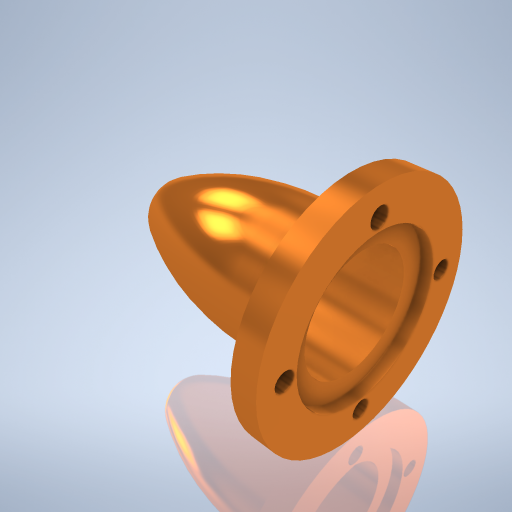
# Autodesk Inventor part: heizrohr
Saved by Autodesk Inventor 2024.2 (Build 282272000, 272)
## iProperties
Created: 2024-04-15
Part Number: heizrohr
Material: Gold
Document SubType Name: Modeling
Designer: Fabri
Density: 19.3 g/cm^3
Appearance: Metall - 1600F (heiß)
Author: Fabri
Autodesk Inventor part; units mm, degrees
ref_plane "YZ Plane" through (0, 0, 0) normal (1, 0, 0) x (0, 1, 0)
ref_plane "XY Plane" through (0, 0, 0) normal (0, 0, 1) x (1, 0, 0)
sketch "Skizze2" plane through (0, 0, 0) normal (0, 0, 1) x (1, 0, 0)
  line L0 (0, 0) -> (39, 0)
  arc A0 (3.1317, 5.27) -> (0, 0) centre (6, 0) ccw
  arc A1 (25.6458, 11) -> (3.1317, 5.27) centre (25.6458, -36.0959) ccw
  line L1 (25.6458, 11) -> (35, 11)
  line L2 (35, 11) -> (35, 19.5)
  line L3 (35, 19.5) -> (39, 19.5)
  line L4 (39, 19.5) -> (39, 0)
  dimension "d12" = 39
  dimension "d13" = 4
  dimension "d14" = 22
  dimension "d15" = 39
  dimension "d16" = 33
  dimension "d17" = 10.54
  dimension "d18" = 36.0959
  constraints: 10 end point, 4 point on circle, 3 perpendicular, 2 centre point, 2 horizontal, 2 tangent, 1 point on line
  measures "d12" distance of L0.start L0.end
  measures "d13" distance between parallel lines of L4 L2
  measures "d14" diameter of L1.start L0
  measures "d15" diameter of L3 L0
  measures "d16" distance from line of L4 A0.centre
  measures "d17" diameter of A0.start L0
  measures "d18" vertical distance of L0.start A1.centre
revolve "Umdrehung2" add sketch "Skizze2" angle 360 about axis through (0, 0, 0) along (1, 0, 0)
ref_plane "Arbeitsebene1" through (0, 0, 0) normal (0, 1, 0) x (-1, 0, 0)
sketch "Skizze3" plane through (0, 0, 0) normal (0, 1, 0) x (-1, 0, 0)
  arc A0 (-25.6458, -11) -> (-3.1317, -5.27) centre (-25.6458, 36.0959) ccw projected
  line L0 (-25.6458, -11) -> (-35, -11) projected
  arc A1 (-3.1317, -5.27) -> (-3.1317, 5.27) centre (-6, 0) ccw projected
  line L1 (-3.1317, 5.27) -> (-3.1317, -5.27) projected
  arc A2 (-3.1317, -3.95) -> (-0.7875, 0) centre (-5.2875, 0) ccw
  arc A3 (-25.9348, -9.5) -> (-3.1317, -3.95) centre (-24.9293, 35.9889) ccw
  line L2 (-25.9348, -9.5) -> (-34.7728, -9.5)
  line L3 (-34.7728, -9.5) -> (-39, -9.5)
  line L4 (-39, 19.5) -> (-39, -19.5) projected
  line L5 (0, 0) -> (-41.9198, 0)
  point P0 (-3.1317, 0)
  point P1 (-39, 0)
  dimension "d22" = 7.9
  dimension "d23" = 4.5
  dimension "d24" = 45.5
  dimension "d25" = 19
  constraints: 6 end point, 5 point on circle, 3 point on line, 2 centre point, 2 horizontal, 2 horizontal alignment, 1 tangent
  measures "d22" diameter of A2.start L5
  measures "d23" radius of A2
  measures "d24" radius of A3
  measures "d25" diameter of L3.end L5
revolve "Umdrehung3" cut sketch "Skizze3" angle 360 about axis through (0, 0, 0) along (1, 0, 0) contours A3 L2 L3 L4 L5 L1
sketch "Skizze4" plane through (39, 0, 0) normal (1, 0, 0) x (0, 0, -1)
  point P0 (0, 0)
  point P1 (0, -15)
  dimension "d27" = 15
  constraints: 1 vertical alignment
  measures "d27" distance of point (0, 0) point (0, -15)
hole "Bohrung1" at (39, -15, 0) direction (-1, 0, 0) diameter 3.2 depth 4
pattern_circular "Runde Anordnung1" count 4 over 360 about axis through (37, 0, 0) along (1, 0, 0) of "Bohrung1"
sketch "Skizze5" plane through (39, 0, 0) normal (1, 0, 0) x (0, 0, -1)
  circle A0 centre (0, 0) radius 13
  dimension "d38" = 26
  constraints: 1 centre point, 1 coincident
  measures "d38" diameter of A0
extrude "Extrusion1" cut sketch "Skizze5" against normal blind 2
